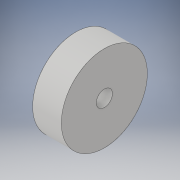
# Autodesk Inventor part: Pretend it's a Flywheel
Saved by Autodesk Inventor 2018 (Build 220112000, 112)
## iProperties
Created: 2020-02-18
Part Number: Pretend it's a Flywheel
Material: Generic
Document SubType Name: Modeling
Designer: T3500STATIC
Density: 1 g/cm^3
Appearance: Default
Author: T3500STATIC
Autodesk Inventor part; units mm, degrees
ref_plane "YZ Plane" through (0, 0, 0) normal (1, 0, 0) x (0, 1, 0)
ref_plane "XZ Plane" through (0, 0, 0) normal (0, 1, 0) x (-1, 0, 0)
ref_plane "XY Plane" through (0, 0, 0) normal (0, 0, 1) x (1, 0, 0)
sketch "Sketch1" plane through (0, 0, 0) normal (1, 0, 0) x (0, 1, 0)
  circle A0 centre (0, 0) radius 76.2
  circle A1 centre (0, 0) radius 14.2875
  dimension "d0" = 152.4
  dimension "d1" = 28.575
  constraints: 2 centre point, 2 coincident
  measures "d0" diameter of A0
  measures "d1" diameter of A1
extrude "Extrusion1" add sketch "Sketch1" along normal blind 50.8
body "Solid1"
